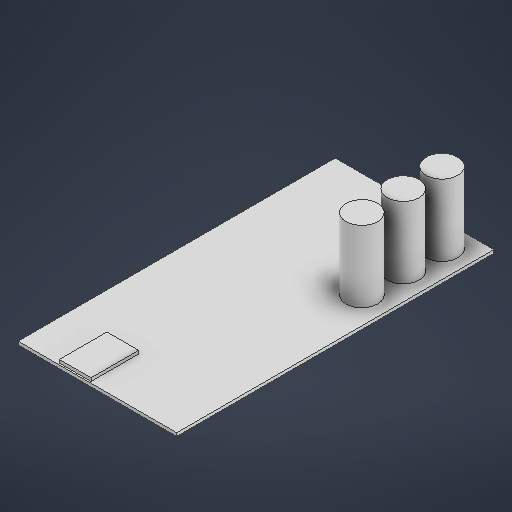
# Autodesk Inventor part: modelo placa
Saved by Autodesk Inventor 2026.2 (Build 302298010, 298A)
## iProperties
Created: 2026-03-05
Part Number: modelo placa
Material: Generic
Document SubType Name: Sheet Metal
Designer: trini
Density: 1 g/cm^3
Sheet Metal Rule: Default
Appearance: Default
Author: trini
Autodesk Inventor part; units mm, degrees
ref_plane "YZ Plane" through (0, 0, 0) normal (1, 0, 0) x (0, 1, 0)
ref_plane "XZ Plane" through (0, 0, 0) normal (0, 1, 0) x (-1, 0, 0)
ref_plane "XY Plane" through (0, 0, 0) normal (0, 0, 1) x (1, 0, 0)
sketch "Sketch2" plane through (0, 0, 0) normal (0, 1, 0) x (-1, 0, 0)
  line L0 (-50, -100) -> (50, -100)
  line L1 (50, -100) -> (50, 100)
  line L2 (50, 100) -> (-50, 100)
  line L3 (-50, 100) -> (-50, -100)
  line L4 (-50, -100) -> (50, 100) construction
  line L5 (50, -100) -> (-50, 100) construction
  point P0 (0, 0)
  dimension "d0" = 200
  dimension "d1" = 100
  constraints: 12 end point, 2 midpoint, 2 parallel, 1 horizontal, 1 perpendicular
  measures "d0" distance of L0.end L1.end
  measures "d1" distance of L0.start L0.end
extrude "Extrusion1" add sketch "Sketch2" along normal blind 2
sketch "Sketch3" plane through (0, 2, 0) normal (0, 1, 0) x (1, 0, 0)
  circle A0 centre (33.1152, 84.1449) radius 10
  circle A1 centre (33.1152, 59.7195) radius 10
  circle A2 centre (33.1152, 33.634) radius 10
  point P0 (0, 0)
  dimension "d4" = 20
  dimension "d5" = 20
  dimension "d6" = 20
  constraints: 3 centre point
  measures "d4" diameter of A0
  measures "d5" diameter of A1
  measures "d6" diameter of A2
extrude "Extrusion2" add sketch "Sketch3" along normal blind 45
sketch "Sketch4" plane through (0, 2, 0) normal (0, 1, 0) x (1, 0, 0)
  line L0 (-25, -99) -> (-5, -99)
  line L1 (-5, -99) -> (-5, -69)
  line L2 (-5, -69) -> (-25, -69)
  line L3 (-25, -69) -> (-25, -99)
  line L4 (-25, -99) -> (-5, -69) construction
  line L5 (-5, -99) -> (-25, -69) construction
  line L6 (-50, 100) -> (-50, -100) projected
  line L7 (-50, -100) -> (50, -100) projected
  point P0 (0, 0)
  point P1 (-15, -84)
  dimension "d9" = 25
  dimension "d10" = 45
  dimension "d11" = 30
  dimension "d12" = 1
  constraints: 12 end point, 2 midpoint, 2 parallel, 1 horizontal, 1 perpendicular
  measures "d9" distance between parallel lines of L6 L3
  measures "d10" distance between parallel lines of L1 L6
  measures "d11" distance between parallel lines of L2 L0
  measures "d12" distance between parallel lines of L7 L0
extrude "Extrusion3" add sketch "Sketch4" along normal blind 2
equation "\"BendRadius\" = Thickness"
equation "\"BendReliefWidth\" = Thickness"
equation "\"BendReliefDepth\" = 0.5 * Thickness"
equation "\"CornerReliefSize\" = 4 * Thickness"
equation "\"MinimumRemnant\" = 2 * Thickness"
equation "\"TransitionRadius\" = BendRadius"
equation "\"JacobiRadiusSize\" = BendRadius"
equation "\"GapSize\" = Thickness"
equation "\"Thickness\" = 3.048"
body "Solid1"
